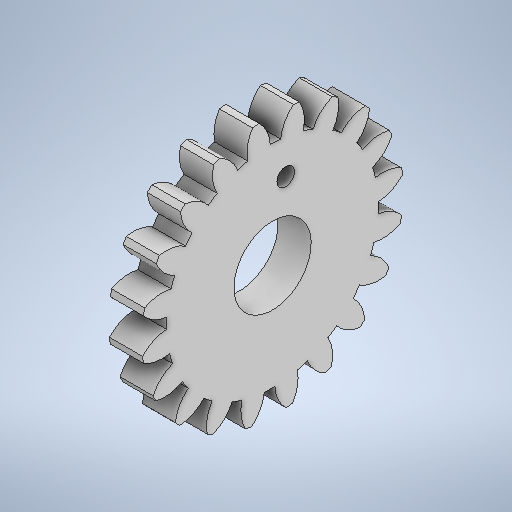
# Autodesk Inventor part: engrane_v5
Saved by Autodesk Inventor 2025.2 (Build 292293000, 293)
## iProperties
Created: 2025-03-05
Part Number: engrane_v5
Material: Generic
Document SubType Name: Modeling
Designer: cdavi
Density: 1 g/cm^3
Appearance: Default
Author: cdavi
Autodesk Inventor part; units mm, degrees
ref_plane "YZ Plane" through (0, 0, 0) normal (1, 0, 0) x (0, 1, 0)
ref_plane "XZ Plane" through (0, 0, 0) normal (0, 1, 0) x (-1, 0, 0)
ref_plane "XY Plane" through (0, 0, 0) normal (0, 0, 1) x (1, 0, 0)
sketch "Sketch1" plane through (0, 0, 0) normal (1, 0, 0) x (0, 1, 0)
  circle A0 centre (0, 0) radius 3.5
  line L0 (0, 0) -> (-3.5, 0)
  circle A1 centre (0, 0) radius 10.7889 construction
  circle A2 centre (0, 0) radius 9.6
  circle A3 centre (0, 0) radius 11.851 construction
  arc A4 (9.5711, -0.7449) -> (9.6, 0) centre (0, 0) ccw
  arc A5 (9.1927, -2.7667) -> (9.5711, -0.7449) centre (0, 0) ccw construction
  line L1 (9.4362, -1.7659) -> (11.6488, -2.18) construction
  arc A6 (11.592, -2.464) -> (11.6986, -1.8948) centre (0, 0) ccw
  arc A7 (11.6986, -1.8948) -> (9.5711, -0.7449) centre (9.2261, -3.9262) ccw
  arc A8 (9.1927, -2.7667) -> (11.592, -2.464) centre (10.0215, 0.3241) ccw
  line L2 (0, 0) -> (11.6488, -2.18) construction
  circle A9 centre (6.3891, -1.1957) radius 0.8
  dimension "d17" = 7
  dimension "d32" = 4.45
  dimension "d34" = 12.3
  dimension "d36" = 3.2
  dimension "d37" = 2.8
  dimension "d42" = 1.1888
  dimension "d43" = 1.0621
  dimension "d45" = 2.3
  dimension "d46" = 1.6
  dimension "d47" = 6.5
  constraints: 18 point on circle, 9 centre point, 7 coincident, 6 end point, 3 concentric, 2 horizontal alignment, 1 horizontal, 1 line through centre, 1 point on line, 1 symmetric about line, 4 other
  measures "d36" radius of A7
  measures "d42" radial gap between concentric circles of A1 A2
  measures "d43" radial gap between concentric circles of A3 A1
  measures "d46" diameter of A9
  measures "d47" distance of A9.centre point (0, 0)
extrude "Extrusion1" add sketch "Sketch1" along normal blind 3 contours A2
extrude "Extrusion3" add sketch "Sketch1" along normal blind 3 contours A2 A7 A6 A8
pattern_circular "Circular Pattern2" count 20 over 360 about axis through (-10, 0, 0) along (1, 0, 0) of "Extrusion3"
equation "\"d17\" = d_agu"
equation "\"d_agu\" = 7"
body "Solid1"
